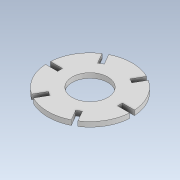
# Autodesk Inventor part: Ring_n7
Saved by Autodesk Inventor 2020 (Build 240168000, 168)
## iProperties
Created: 2020-09-11
Part Number: Ring_n7
Material: Generic
Document SubType Name: Modeling
Designer: Admin
Density: 1 g/cm^3
Appearance: Default
Author: Admin
Autodesk Inventor part; units mm, degrees
ref_plane "YZ Plane" through (0, 0, 0) normal (1, 0, 0) x (0, 1, 0)
ref_plane "XZ Plane" through (0, 0, 0) normal (0, 1, 0) x (-1, 0, 0)
ref_plane "XY Plane" through (0, 0, 0) normal (0, 0, 1) x (1, 0, 0)
sketch "Sketch1" plane through (0, 0, 0) normal (0, 1, 0) x (-1, 0, 0)
  circle A0 centre (0, 0) radius 17.325
  circle A1 centre (0, 0) radius 7.325
  dimension "d0" = 34.65
  dimension "d1" = 14.65
  constraints: 2 centre point, 2 coincident
  measures "d0" diameter of A0
  measures "d1" diameter of A1
extrude "Extrusion1" add sketch "Sketch1" along normal blind 2
sketch "Sketch2" plane through (0, 2, 0) normal (0, 1, 0) x (1, 0, 0)
  line L0 (-22.325, -1) -> (-12.325, -1)
  line L1 (-12.325, -1) -> (-12.325, 1)
  line L2 (-12.325, 1) -> (-22.325, 1)
  line L3 (-22.325, 1) -> (-22.325, -1)
  point P0 (0, 0)
  dimension "d4" = 1
  dimension "d5" = 2
  dimension "d6" = 12.325
  dimension "d7" = 10
  constraints: 8 end point, 2 parallel, 1 horizontal, 1 perpendicular
  measures "d4" distance from line of point (0, 0) L0
  measures "d5" distance of L2.end L0.start
  measures "d6" distance from line of point (0, 0) L1
  measures "d7" distance of L1.end L2.end
extrude "Extrusion2" cut sketch "Sketch2" against normal blind 2
pattern_circular "Circular Pattern2" count 6 over 360 about axis through (0, -10, 0) along (0, 1, 0) of "Extrusion2"
body "Solid1"
